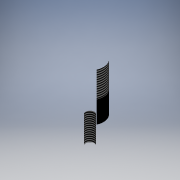
# Autodesk Inventor part: Spigot Long
Saved by Autodesk Inventor 2019 (Build 230136000, 136)
## iProperties
Created: 2016-04-18
Part Number: Spigot Long
Material: Aluminum 6061
Document SubType Name: Modeling
Designer: IEUser
Density: 2.7 g/cm^3
Appearance: Anodized - Black
Author: IEUser
Autodesk Inventor part; units mm, degrees
ref_plane "YZ Plane" through (0, 0, 0) normal (1, 0, 0) x (0, 1, 0)
ref_plane "XZ Plane" through (0, 0, 0) normal (0, 1, 0) x (-1, 0, 0)
ref_plane "XY Plane" through (0, 0, 0) normal (0, 0, 1) x (1, 0, 0)
sketch "Spigot Base Outline" plane through (0, 0, 0) normal (0, 1, 0) x (-1, 0, 0)
  line L0 (-8, -5.1235) -> (-8, 5.1235)
  line L1 (8, 5.1235) -> (8, -5.1235)
  arc A0 (-8, -5.1235) -> (8, -5.1235) centre (0, 0) ccw
  arc A1 (8, 5.1235) -> (-8, 5.1235) centre (0, 0) ccw
  dimension "d1" = 9.5
  dimension "d2" = 9.5
  dimension "d3" = 8
  dimension "d4" = 8
  constraints: 4 end point, 4 point on circle, 2 centre point, 1 coincident, 1 parallel, 1 vertical
  measures "d1" radius of A0
  measures "d2" radius of A1
  measures "d3" distance from line of point (0, 0) L1
  measures "d4" distance from line of point (0, 0) L0
extrude "Spigot Base" add sketch "Spigot Base Outline" against normal blind 10
sketch "Spigot Cross Section" plane through (0, 0, 0) normal (0, 1, 0) x (1, 0, 0)
  circle A0 centre (0, 0) radius 4.95
  dimension "d7" = 9.9
  constraints: 1 centre point, 1 coincident
  measures "d7" diameter of A0
extrude "Spigot" add sketch "Spigot Cross Section" along normal blind 25.5
sketch "Clip Cutout Profile" plane through (0, 0, 0) normal (0, 0, 1) x (1, 0, 0)
  line L0 (7.707, 25.5) -> (4.25, 25.5)
  line L1 (4.25, 25.5) -> (4.25, 22.4178)
  line L2 (4.25, 22.4178) -> (2.8322, 21)
  line L3 (2.8322, 21) -> (4.25, 19.5822)
  line L4 (4.25, 19.5822) -> (4.25, 17.5)
  line L5 (4.25, 17.5) -> (7.707, 17.5)
  line L6 (7.707, 17.5) -> (7.707, 25.5)
  circle A0 centre (4.6, 21) radius 1.25 construction
  line L7 (4.95, 25.5) -> (-4.95, 25.5) projected
  line L8 (0, -17.1) -> (0, 32.6) projected
  point P0 (0, 0)
  dimension "d10" = 45
  dimension "d11" = 45
  dimension "d12" = 2.5
  dimension "d13" = 0
  dimension "d15" = 8
  dimension "d16" = 3.457
  dimension "d17" = 4.6
  dimension "d18" = 4.5
  dimension "d19" = 4.25
  constraints: 14 end point, 3 perpendicular, 2 tangent, 1 centre point, 1 collinear, 1 horizontal
  measures "d10" angle of L1 L2
  measures "d11" angle of L4 L3
  measures "d12" diameter of A0
  measures "d13" distance between parallel lines of L0 L7
  measures "d15" distance of L5.end L0.start
  measures "d16" distance of L0.start L0.end
  measures "d17" horizontal distance of point (0, 0) A0.centre
  measures "d18" distance from line of L0 A0.centre
  measures "d19" distance from line of point (0, 0) L1
revolve "Clip Cutout" cut sketch "Clip Cutout Profile" angle 360 about axis through (0, 0, 0) along (0, 1, 0)
thread "Thread" size "M10x0.75" class "6g" standard "ANSI Metric M Profile" length 9.5
hole "Connector Hole" at (0, 25.5, 0) direction (0, -1, 0) diameter 4.826 depth 25 tip angle 118 counterbore diameter 6.477 counterbore depth 2.032
sketch "Orientation Cutout Profile" plane through (0, 25.5, 0) normal (0, 1, 0) x (1, 0, 0)
  arc A0 (-2.0382, -4.5109) -> (-2.0382, 4.5109) centre (0, 0) ccw
  line L0 (-3.95, 1.5492) -> (-3.95, -1.5492)
  arc A1 (-2.0382, 4.5109) -> (-3.95, 1.5492) centre (-0.7, 1.5492) ccw
  arc A2 (-3.95, -1.5492) -> (-2.0382, -4.5109) centre (-0.7, -1.5492) ccw
  line L1 (-10, 10) -> (10, 10)
  line L2 (10, 10) -> (10, -10)
  line L3 (10, -10) -> (-10, -10)
  line L4 (-10, -10) -> (-10, 10)
  point P0 (0, 0)
  point P1 (-3.95, 2.9833)
  point P2 (-3.95, -2.9833)
  dimension "d38" = 4.95
  dimension "d39" = 3.95
  dimension "d40" = 3.25
  dimension "d41" = 20
  dimension "d42" = 10
  dimension "d43" = 20
  dimension "d44" = 10
  constraints: 10 end point, 8 point on circle, 4 tangent, 3 centre point, 2 parallel, 2 point on line, 1 coincident, 1 equal radius, 1 horizontal, 1 perpendicular, 1 vertical
  measures "d38" radius of A0
  measures "d39" distance from line of point (0, 0) L0
  measures "d40" radius of A1
  measures "d41" distance of L1.start L1.end
  measures "d42" distance from line of point (0, 0) L4
  measures "d43" distance of L3.end L1.start
  measures "d44" distance from line of point (0, 0) L1
extrude "Orientation Cutout" cut sketch "Orientation Cutout Profile" against normal blind 25.5
sketch "Cable Hole Position" plane through (-3.95, 0, -1.5492) normal (-1, 0, 0) x (0, 0, 1)
  line L0 (0, 25.5) -> (3.0984, 25.5) projected
  point P0 (1.5492, 0)
  point P1 (1.5492, 4.5)
  point P2 (0.1203, 25.5)
  point P3 (2.9926, 25.5)
  dimension "d47" = 0
  dimension "d48" = 21
  measures "d47" horizontal distance of point (1.549, 4.5) point (1.549, 0)
  measures "d48" distance from line of L0 point (1.549, 4.5)
hole "Cable Hole" at (-3.95, 4.5, 0) direction (1, 0, 0) diameter 4.826 depth 4
chamfer "Top Chamfer" distance 0.254 angle 45 2 edges at (0, 23.468, -2.413) (4.25, 25.5, 0)
chamfer "Bottom Chamfer" distance 1 angle 45 2 edges at (0, -10, 9.5) (0, -10, -9.5)
hole "Connector Box Fastening Hole" at (0, -10, 0) direction (0, 1, 0) diameter 3.242 depth 11.8 tip angle 118 thread size "M4x0.7" class "6H" standard "ISO Metric profile"
equation "\"d2\" = d1"
equation "\"d4\" = d3"
equation "\"d38\" = 0.5 * d7"
equation "\"d42\" = 0.5 * d41"
equation "\"d44\" = 0.5 * d43"
body "Solid1"
